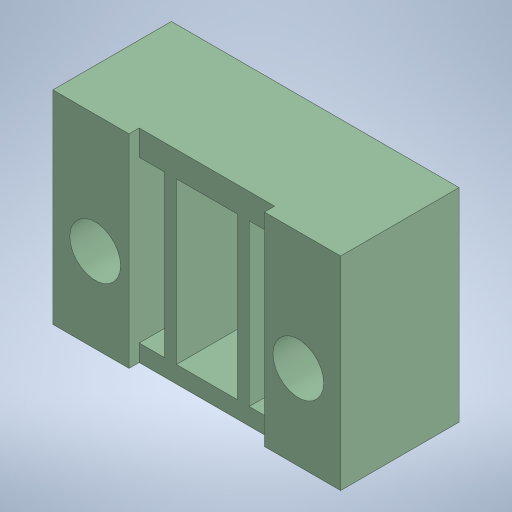
# Autodesk Inventor part: greiper_TPU
Saved by Autodesk Inventor 2024 (Build 280153000, 153)
## iProperties
Created: 2025-06-13
Part Number: greiper_TPU
Material: ゴム、シリコーン
Document SubType Name: Modeling
Designer: 1412z
Density: 1.25 g/cm^3
Appearance: ゴム - 緑
Author: 1412z
Autodesk Inventor part; units mm, degrees
ref_plane "YZ Plane" through (0, 0, 0) normal (1, 0, 0) x (0, 1, 0)
ref_plane "XZ Plane" through (0, 0, 0) normal (0, 1, 0) x (-1, 0, 0)
ref_plane "XY Plane" through (0, 0, 0) normal (0, 0, 1) x (1, 0, 0)
sketch "スケッチ1" plane through (0, 0, 0) normal (0, 0, 1) x (1, 0, 0)
  line L0 (8.5, 7) -> (-8.5, 7)
  line L1 (-8.5, 7) -> (-8.5, -7)
  line L2 (-8.5, -7) -> (8.5, -7)
  line L3 (8.5, -7) -> (8.5, 7)
  line L4 (8.5, 7) -> (-8.5, -7) construction
  line L5 (-8.5, 7) -> (8.5, -7) construction
  circle A0 centre (-6, -2) radius 1.5
  circle A1 centre (6, -2) radius 1.5
  line L6 (-8.5, -6) -> (8.5, -6)
  line L7 (-8.5, 3.5) -> (8.5, 3.5)
  line L8 (-4, -7) -> (-4, 7)
  line L9 (4, -7) -> (4, 7)
  line L10 (2.5, -6) -> (2.5, 3.5)
  line L11 (-2.5, -6) -> (-2.5, 3.5)
  line L12 (1.8, -6) -> (1.8, 3.5)
  line L13 (-1.8, -6) -> (-1.8, 3.5)
  point P0 (0, 0)
  point P1 (-4, -6)
  point P2 (-4, 3.5)
  point P3 (4, -6)
  point P4 (4, 3.5)
  dimension "d0" = 17
  dimension "d1" = 14
  dimension "d2" = 3
  dimension "d3" = 3
  dimension "d4" = 3.5
  dimension "d5" = 4.5
  dimension "d6" = 4.5
  dimension "d7" = 1.5
  dimension "d8" = 1.5
  dimension "d9" = 1
  dimension "d16" = 0.7
  dimension "d17" = 0.7
  dimension "d22" = 5
  dimension "d23" = 5
  constraints: 28 end point, 16 point on line, 9 perpendicular, 2 centre point, 2 midpoint, 2 parallel, 1 horizontal
  measures "d0" distance of L2.end L1.end
  measures "d1" distance of L1.end L0.end
  measures "d2" diameter of A0
  measures "d3" diameter of A1
  measures "d4" distance between parallel lines of L0 L7
  measures "d5" distance between parallel lines of L9 L3
  measures "d6" distance between parallel lines of L1 L8
  measures "d7" distance between parallel lines of L10 L9
  measures "d8" distance between parallel lines of L8 L11
  measures "d9" distance between parallel lines of L2 L6
  measures "d16" distance between parallel lines of L13 L11
  measures "d17" distance between parallel lines of L10 L12
  measures "d22" distance from line of A0.centre L2
  measures "d23" distance from line of A1.centre L2
extrude "押し出し1" add sketch "スケッチ1" along normal blind 7 contours L3 L7 L9 L0 | L9 L7 L8 L0 | L3 L6 L9 L7 | L8 L7 L1 L0 | L3 L2 L9 L6 | L8 L6 L1 L7 | L10 L6 L12 L7 | L9 L2 L8 L6 | L7 L13 L6 L11 | L8 L2 L1 L6
sketch "スケッチ2" plane through (0, 0, 7) normal (0, 0, 1) x (1, 0, 0)
  line L0 (8.5, 7) -> (-8.5, 7) projected
  line L1 (0, 7) -> (-4, 7)
  line L2 (-4, 7) -> (-4, -7)
  line L3 (-8.5, -7) -> (8.5, -7) projected
  line L4 (-4, -7) -> (4, -7)
  line L5 (4, -7) -> (4, 7)
  line L6 (4, 7) -> (0, 7)
  point P0 (0, 0)
  dimension "d12" = 4
  dimension "d13" = 8
  constraints: 10 end point, 4 point on line, 2 perpendicular, 1 collinear, 1 midpoint
  measures "d12" distance of L1.start L1.end
  measures "d13" distance of L2.end L4.end
extrude "押し出し2" cut sketch "スケッチ2" against normal blind 0.6
sketch "スケッチ3" plane through (-8.5, 7, 0) normal (0, 1, 0) x (1, 0, 0)
  line L0 (0, 0) -> (0, -7) projected
  line L1 (17, 0) -> (17, -7) projected
  line L2 (0, 0) -> (17, 0)
  line L3 (17, 0) -> (17, -7)
  line L4 (17, -7) -> (0, -7)
  line L5 (0, -7) -> (0, 0)
  point P0 (8.5, 0)
  point P1 (0, -7)
  constraints: 8 end point, 2 parallel, 1 horizontal, 1 perpendicular
extrude "押し出し3" cut sketch "スケッチ3" against normal blind 2
